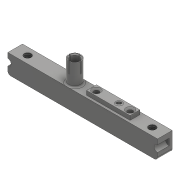
# Autodesk Inventor part: lightBlocker
Saved by Autodesk Inventor 2018 (Build 220112000, 112)
## iProperties
Created: 2017-05-11
Part Number: lightBlocker
Material: ABS Plastic
Document SubType Name: Modeling
Designer: sawaiz
Density: 1.06 g/cm^3
Appearance: Smooth - Medium Gray
Author: sawaiz
Autodesk Inventor part; units mm, degrees
ref_plane "YZ Plane" through (0, 0, 0) normal (1, 0, 0) x (0, 1, 0)
ref_plane "XZ Plane" through (0, 0, 0) normal (0, 1, 0) x (-1, 0, 0)
ref_plane "XY Plane" through (0, 0, 0) normal (0, 0, 1) x (1, 0, 0)
sketch "Sketch1" plane through (0, 0, 0) normal (0, 1, 0) x (-1, 0, 0)
  line L0 (35.7, 4.5) -> (-35.7, 4.5)
  line L1 (-35.7, 4.5) -> (-35.7, -4.5)
  line L2 (-35.7, -4.5) -> (35.7, -4.5)
  line L3 (35.7, -4.5) -> (35.7, 4.5)
  line L4 (35.7, 4.5) -> (-35.7, -4.5) construction
  line L5 (-35.7, 4.5) -> (35.7, -4.5) construction
  point P0 (0, 0)
  dimension "d0" = 71.4
  dimension "d1" = 9
  constraints: 12 end point, 2 midpoint, 2 parallel, 1 horizontal, 1 perpendicular
  measures "d0" distance of L1.end L2.end
  measures "d1" distance of L0.end L1.end
extrude "Extrusion1" add sketch "Sketch1" along normal mid plane 7
sketch "Sketch2" plane through (-35.7, 3.5, 4.5) normal (0, 0, 1) x (1, 0, 0)
  line L0 (0, 0) -> (0, -7) projected
  line L1 (0, -3.5) -> (71.4, -3.5) construction
  line L2 (71.4, -7) -> (71.4, 0) projected
  point P0 (35.7, -3.5)
  point P1 (6, -3.5)
  point P2 (65.4, -3.5)
  dimension "d4" = 6
  dimension "d5" = 65.4
  constraints: 2 end point, 2 midpoint, 2 point on line
  measures "d4" distance from line of L0 point (6, -3.5)
  measures "d5" distance from line of L0 point (65.4, -3.5)
hole "Hole1" at (-29.7, 0, 4.5) at (29.7, 0, 4.5) direction (0, 0, -1) diameter 3.242 depth 8 thread size "M4x0.7" class "6H" standard "ANSI Metric M Profile"
fillet "Fillet1" radius 1.5 2 edges at (35.7, 0, -4.5) (-35.7, 0, -4.5)
sketch "Sketch3" plane through (-35.7, 3.5, 4.5) normal (0, 0, 1) x (1, 0, 0)
  line L0 (0, 0) -> (0, -7) projected
  line L1 (0, -3.5) -> (28.4, -3.5) construction
  point P0 (35.7, -3.5)
  dimension "d14" = 28.4
  constraints: 2 end point, 1 horizontal, 1 midpoint
  measures "d14" distance from line of L0 L1.end
hole "Hole2" at (-7.3, 0, 4.5) direction (0, 0, -1) diameter 4.3 end through all
sketch "Sketch4" plane through (-35.7, 3.5, 4.5) normal (0, 0, 1) x (1, 0, 0)
  circle A0 centre (28.4, -3.5) radius 2.15 projected
  circle A1 centre (28.4, -3.5) radius 2.9
  point P0 (35.7, -3.5)
  dimension "d22" = 5.8
  constraints: 1 centre point, 1 coincident
  measures "d22" diameter of A1
extrude "Extrusion2" add sketch "Sketch4" along normal blind 10.2
sketch "Sketch5" plane through (34.2, 3.5, -4.5) normal (0, 0, -1) x (-1, 0, 0)
  circle A0 centre (41.5, -3.5) radius 2.15 projected
  circle A1 centre (41.5, -3.5) radius 2.25
  point P0 (34.2, -3.5)
  dimension "d25" = 4.5
  constraints: 1 centre point, 1 coincident
  measures "d25" diameter of A1
extrude "Extrusion3" cut sketch "Sketch5" against normal blind 14.3 contours A0 | A1
sketch "Sketch6" plane through (0, -3.5, 0) normal (0, -1, 0) x (1, 0, 0)
  arc A0 (-35.7, -3) -> (-34.2, -4.5) centre (-34.2, -3) ccw projected
  line L0 (-34.2, -4.5) -> (34.2, -4.5) projected
  arc A1 (34.2, -4.5) -> (35.7, -3) centre (34.2, -3) ccw projected
  line L1 (35.7, -3) -> (35.7, 4.5) projected
  line L2 (35.7, 4.5) -> (-35.7, 4.5) projected
  line L3 (-35.7, 4.5) -> (-35.7, -3) projected
  line L4 (-35.7, 4.5) -> (-35.7, -3) projected
  arc A2 (-35.7, -1.1) -> (-35.7, 2.1) centre (-35.7, 0.5) ccw
  line L5 (-35.7, 2.1) -> (-35.7, -1.1)
  point P0 (0, 0)
  dimension "d28" = 1.6
  dimension "d29" = 5
  constraints: 3 point on line, 2 end point, 2 point on circle, 1 centre point, 1 collinear
  measures "d28" radius of A2
  measures "d29" distance from line of L0 A2.centre
extrude "Extrusion4" cut sketch "Sketch6" against normal blind 5.5 contours L3 A2
mirror "Mirror1" about plane through (0, 0, 0) normal (1, 0, 0) of "Extrusion4"
fillet "Fillet2" radius 0.8 1 edges at (-10.2, 0, 4.5)
sketch "Sketch7" plane through (35.7, -3.5, 4.5) normal (0, 0, 1) x (1, 0, 0)
  line L0 (-34.9, 1.1) -> (-14.2, 1.1)
  line L1 (-14.2, 1.1) -> (-14.2, 5.8)
  line L2 (-14.2, 5.8) -> (-34.9, 5.8)
  line L3 (-34.9, 5.8) -> (-34.9, 1.1)
  line L4 (-34.9, 1.1) -> (-14.2, 5.8) construction
  line L5 (-14.2, 1.1) -> (-34.9, 5.8) construction
  line L6 (0, 0) -> (-41.8, 0) projected
  line L7 (-71.4, 7) -> (-71.4, 0) projected
  point P0 (-35.7, 3.5)
  point P1 (-24.55, 3.45)
  dimension "d33" = 1.1
  dimension "d34" = 4.7
  dimension "d35" = 20.7
  dimension "d36" = 36.5
  constraints: 12 end point, 2 midpoint, 2 parallel, 1 horizontal, 1 perpendicular
  measures "d33" distance between parallel lines of L6 L0
  measures "d34" distance of L0.end L1.end
  measures "d35" distance of L1.end L2.end
  measures "d36" distance between parallel lines of L7 L3
extrude "Extrusion5" add sketch "Sketch7" along normal blind 2
sketch "Sketch8" plane through (35.7, -3.5, 6.5) normal (0, 0, 1) x (1, 0, 0)
  line L0 (-34.9, 1.1) -> (-14.2, 1.1) projected
  line L1 (-14.2, 1.1) -> (-14.2, 5.8) projected
  line L2 (-14.2, 5.8) -> (-34.9, 5.8) projected
  line L3 (-34.9, 5.8) -> (-34.9, 1.1) projected
  line L4 (-34.9, 3.45) -> (-14.2, 3.45) construction
  line L5 (-71.4, 7) -> (-71.4, 0) projected
  point P0 (-35.7, 3.5)
  point P1 (-32.6, 3.45)
  point P2 (-16.5, 3.45)
  dimension "d39" = 38.8
  dimension "d40" = 16.1
  constraints: 2 end point, 2 midpoint, 2 point on line
  measures "d39" distance from line of point (-32.6, 3.45) L5
  measures "d40" distance of point (-32.6, 3.45) point (-16.5, 3.45)
hole "Hole3" at (3.1, -0.05, 6.5) at (19.2, -0.05, 6.5) direction (0, 0, -1) diameter 2.4 end through all countersink diameter 3.9 countersink angle 90
sketch "Sketch9" plane through (34.2, 3.5, -4.5) normal (0, 0, -1) x (-1, 0, 0)
  circle A0 centre (31.1, -3.55) radius 1.2 projected
  circle A1 centre (15, -3.55) radius 1.2 projected
  circle A2 centre (41.5, -3.5) radius 2.25 projected
  line L0 (68.4, 0) -> (68.4, -7) projected
  line L1 (0, 0) -> (68.4, 0) projected
  line L2 (0, -7) -> (0, 0) projected
  line L3 (68.4, -7) -> (0, -7) projected
  circle A3 centre (15, -3.55) radius 1.2 projected
  circle A4 centre (15, -3.55) radius 1.45
  circle A5 centre (31.1, -3.55) radius 1.45
  point P0 (34.2, -3.5)
  dimension "d48" = 2.9
  dimension "d49" = 2.9
  constraints: 2 centre point, 2 coincident
  measures "d48" diameter of A4
  measures "d49" diameter of A5
extrude "Extrusion6" cut sketch "Sketch9" against normal blind 8 contours A0 | A1 | A4 | A5
sketch "Sketch11" plane through (0, 0, 0) normal (0, 1, 0) x (-1, 0, 0)
  line L0 (-21.5, 6.5) -> (-0.8, 6.5) projected
  arc A0 (-12.2252, 6.5) -> (-13.8, 6.7) centre (-13.8, 0.4) ccw
  line L1 (-13.8, 6.7) -> (-13.8, 6.5)
  line L2 (-13.8, 6.5) -> (-12.2252, 6.5)
  line L3 (-5.05, 6.5) -> (-1.15, 6.5) projected
  point P0 (0, 0)
  point P1 (-3.1, 6.5)
  dimension "d58" = 6.3
  dimension "d59" = 0.2
  dimension "d60" = 10.7
  constraints: 4 end point, 2 point on circle, 2 point on line, 1 centre point, 1 line through centre, 1 midpoint, 1 perpendicular
  measures "d58" radius of A0
  measures "d59" distance of L1.start L1.end
  measures "d60" distance from line of point (-3.1, 6.5) L1
revolve "Revolution1" add sketch "Sketch11" angle 360 about axis through (13.8, 0, 6.7) along (0, 0, -1)
sketch "Sketch10" plane through (35.7, -3.5, 6.5) normal (0, 0, 1) x (1, 0, 0)
  arc A0 (-21.1222, 3.3793) -> (-21.9707, 4.2278) centre (-21.5464, 3.8036) ccw
  arc A1 (-22.6778, 3.5207) -> (-21.8293, 2.6722) centre (-22.2536, 3.0964) ccw
  line L0 (-21.8293, 2.6722) -> (-21.1222, 3.3793)
  line L1 (-22.6778, 3.5207) -> (-21.9707, 4.2278)
  line L2 (-22.3243, 3.8743) -> (-21.4757, 3.0257) construction
  circle A2 centre (-32.6, 3.45) radius 1.2 projected
  circle A3 centre (-16.5, 3.45) radius 1.2 projected
  line L3 (-32.6, 3.45) -> (-16.5, 3.45) construction
  line L4 (-34.9, 1.1) -> (-14.2, 1.1) projected
  point P0 (-35.7, 3.5)
  point P1 (-21.9, 3.45)
  dimension "d52" = 0.6
  dimension "d53" = 0.6
  dimension "d54" = 10.7
  dimension "d55" = 45
  dimension "d62" = 0.5
  dimension "d63" = 1
  constraints: 8 end point, 4 point on circle, 3 midpoint, 2 centre point, 2 tangent, 1 horizontal, 1 parallel, 1 point on line
  measures "d52" radius of A0
  measures "d53" radius of A1
  measures "d54" distance of L3.start point (-21.9, 3.45)
  measures "d55" angle of L4 L0
  measures "d62" distance of point (-21.9, 3.45) A1.centre
  measures "d63" distance of A0.centre A1.centre
extrude "Extrusion7" cut sketch "Sketch10" along normal through all both and the other way through all contours L0 A1 L1 A0
chamfer "Chamfer1" distance 0.4 angle 45 1 edges at (-9.45, 0, 14.7)
sketch "Sketch12" plane through (-7.3, 0, 14.7) normal (0, 0, 1) x (1, 0, 0)
  line L0 (-0.254, -2.9) -> (0.254, -2.9)
  line L1 (0.254, -2.9) -> (0.254, 2.9)
  line L2 (0.254, 2.9) -> (-0.254, 2.9)
  line L3 (-0.254, 2.9) -> (-0.254, -2.9)
  line L4 (-0.254, -2.9) -> (0.254, 2.9) construction
  line L5 (0.254, -2.9) -> (-0.254, 2.9) construction
  circle A0 centre (0, 0) radius 2.9 projected
  line L6 (-2.9, -0.254) -> (2.9, -0.254)
  line L7 (2.9, -0.254) -> (2.9, 0.254)
  line L8 (2.9, 0.254) -> (-2.9, 0.254)
  line L9 (-2.9, 0.254) -> (-2.9, -0.254)
  line L10 (-2.9, -0.254) -> (2.9, 0.254) construction
  line L11 (2.9, -0.254) -> (-2.9, 0.254) construction
  point P0 (7.3, 0)
  point P1 (0, 0)
  dimension "d64" = 0.508
  dimension "d67" = 0.508
  constraints: 24 end point, 5 midpoint, 4 parallel, 2 horizontal, 2 perpendicular, 2 tangent, 1 coincident
  measures "d64" distance of L1.end L2.end
  measures "d67" distance of L6.end L7.end
extrude "Extrusion8" cut sketch "Sketch12" against normal blind 5.1 contours L3 A0 L0 | A0 L1 L0 | A0 L3 L6 L1 | L6 A0 L8 L3 | L3 L8 L1 L6 | L6 L9 A0 | L1 L8 A0 L6 | A0 L7 L6 | L3 A0 L1 L8 | L9 L8 A0 | A0 L8 L7 | L3 L2 A0 | A0 L2 L1
equation "\"d67\" = d64"
body "Solid1"
